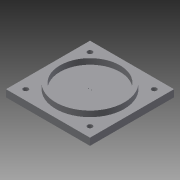
# Autodesk Inventor part: Power_Meter_Adapter_Part2
Saved by Autodesk Inventor 2015 (Build 190159000, 159)
## iProperties
Created: 2015-02-18
Part Number: Power_Meter_Adapter_Part2
Material: Generic
Document SubType Name: Modeling
Designer: sgneitin
Density: 1 g/cm^3
Appearance: Default
Author: sgneitin
Autodesk Inventor part; units mm, degrees
ref_plane "YZ Plane" through (0, 0, 0) normal (1, 0, 0) x (0, 1, 0)
ref_plane "XZ Plane" through (0, 0, 0) normal (0, 1, 0) x (-1, 0, 0)
ref_plane "XY Plane" through (0, 0, 0) normal (0, 0, 1) x (1, 0, 0)
sketch "Sketch1" plane through (0, 0, 0) normal (0, 1, 0) x (-1, 0, 0)
  line L0 (29.75, 29.75) -> (-29.75, 29.75)
  line L1 (-29.75, 29.75) -> (-29.75, -29.75)
  line L2 (-29.75, -29.75) -> (29.75, -29.75)
  line L3 (29.75, -29.75) -> (29.75, 29.75)
  line L4 (29.75, 0) -> (-29.75, 0) construction
  line L5 (0, -29.75) -> (0, 29.75) construction
  circle A0 centre (-22.75, 22.75) radius 1.75
  circle A1 centre (-22.75, -22.75) radius 1.75
  circle A2 centre (22.75, -22.75) radius 1.75
  circle A3 centre (22.75, 22.75) radius 1.75
  circle A4 centre (-1, 0) radius 0.25
  circle A5 centre (1, 0) radius 0.25
  point P0 (0, 0)
  dimension "d0" = 59.5
  dimension "d3" = 3.5
  dimension "d4" = 7
  dimension "d5" = 7
  dimension "d10" = 1
  dimension "d11" = 0.5
  constraints: 12 end point, 6 centre point, 6 midpoint, 4 equal radius, 4 symmetric about line, 2 parallel, 2 perpendicular, 1 horizontal, 1 point on line
  measures "d0" distance of L0.start L0.end
  measures "d3" diameter of A0
  measures "d4" distance from line of L0 A3.centre
  measures "d5" distance from line of L3 A3.centre
  measures "d10" distance from line of A4.centre L5
  measures "d11" diameter of A4
extrude "Extrusion1" add sketch "Sketch1" along normal blind 5
sketch "Sketch3" plane through (0, 5, 0) normal (0, 1, 0) x (1, 0, 0)
  circle A0 centre (0, 0) radius 24.25
  circle A1 centre (0, 0) radius 21.25
  line L0 (29.75, 29.75) -> (-29.75, 29.75) projected
  dimension "d7" = 3
  dimension "d12" = 5.5
  constraints: 2 centre point, 1 coincident, 1 concentric
  measures "d7" radial gap between concentric circles of A0 A1
  measures "d12" distance edge to line of A0 L0
extrude "Extrusion2" add sketch "Sketch3" along normal blind 4
body "Solid1"
